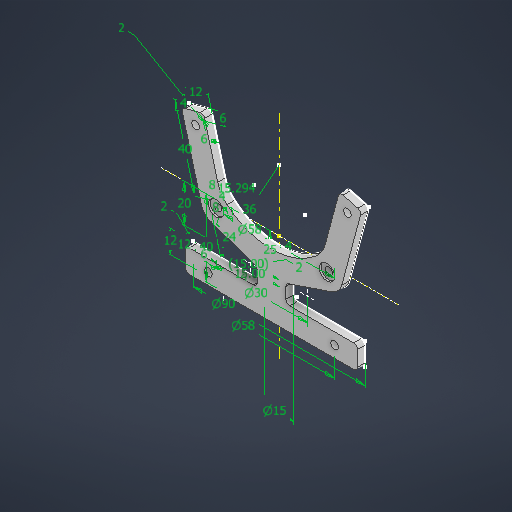
# Autodesk Inventor part: UnitreeGO2_frontmount
Saved by Autodesk Inventor 2026.1 (Build 301233000, 233)
## iProperties
Created: 2026-01-16
Part Number: UnitreeGO2_frontmount
Material: Generic
Document SubType Name: Modeling
Designer: aimot
Density: 1 g/cm^3
Appearance: Default
Author: aimot
Autodesk Inventor part; units mm, degrees
ref_plane "YZ Plane" through (0, 0, 0) normal (1, 0, 0) x (0, 1, 0)
ref_plane "XZ Plane" through (0, 0, 0) normal (0, 1, 0) x (-1, 0, 0)
ref_plane "XY Plane" through (0, 0, 0) normal (0, 0, 1) x (1, 0, 0)
sketch "Sketch1" plane through (0, 0, 0) normal (0, 0, 1) x (1, 0, 0)
  circle A0 centre (-29, 0) radius 2
  line L0 (-62.2888, 0) -> (62.2888, 0) construction
  arc A1 (-36.7274, -2.0706) -> (-31.5768, -7.5737) centre (-29, 0) ccw
  arc A2 (-23.2301, 4.498) -> (0, -4) centre (0, 32) ccw
  line L1 (0, -55.9324) -> (0, 55.5944) construction
  line L2 (-31.5768, -7.5737) -> (-8.8558, -15.304)
  line L3 (-7.5, -17.1974) -> (-7.5, -23)
  line L4 (-36.7274, -2.0706) -> (-46.5625, 34.6346)
  line L5 (-45.1483, 37.0841) -> (-37.4209, 39.1547)
  line L6 (-34.9714, 37.7405) -> (-28.1342, 12.2236)
  arc A3 (-7.5, -17.1974) -> (-8.8558, -15.304) centre (-9.5, -17.1974) ccw
  arc A4 (-45.1483, 37.0841) -> (-46.5625, 34.6346) centre (-44.6307, 35.1523) ccw
  arc A5 (-34.9714, 37.7405) -> (-37.4209, 39.1547) centre (-36.9033, 37.2228) ccw
  circle A6 centre (29, 0) radius 2
  line L7 (62.2888, 0) -> (-62.2888, 0) construction
  arc A7 (31.5768, -7.5737) -> (36.7274, -2.0706) centre (29, 0) ccw
  line L8 (31.5768, -7.5737) -> (8.8558, -15.304)
  line L9 (7.5, -17.1974) -> (7.5, -25)
  line L10 (36.7274, -2.0706) -> (46.5625, 34.6346)
  line L11 (45.1483, 37.0841) -> (37.4209, 39.1547)
  arc A8 (8.8558, -15.304) -> (7.5, -17.1974) centre (9.5, -17.1974) ccw
  arc A9 (46.5625, 34.6346) -> (45.1483, 37.0841) centre (44.6307, 35.1523) ccw
  arc A10 (37.4209, 39.1547) -> (34.9714, 37.7405) centre (36.9033, 37.2228) ccw
  circle A11 centre (-29, 0) radius 4
  circle A12 centre (29, 0) radius 4
  line L12 (-9.5, -25) -> (-43, -25)
  line L13 (-45, -27) -> (-45, -35)
  line L14 (-43, -37) -> (0, -37)
  arc A13 (-43, -25) -> (-45, -27) centre (-43, -27) ccw
  arc A14 (-45, -35) -> (-43, -37) centre (-43, -35) ccw
  arc A15 (-9.5, -25) -> (-7.5, -23) centre (-9.5, -23) ccw
  line L15 (9.5, -25) -> (43, -25)
  line L16 (45, -27) -> (45, -35)
  line L17 (43, -37) -> (0, -37)
  arc A16 (45, -27) -> (43, -25) centre (43, -27) ccw
  arc A17 (43, -37) -> (45, -35) centre (43, -35) ccw
  arc A18 (7.5, -23) -> (9.5, -25) centre (9.5, -23) ccw
  arc A19 (-28.1342, 12.2236) -> (-23.2301, 4.498) centre (-13.3609, 16.1821) ccw
  arc A20 (0, -4) -> (23.2301, 4.498) centre (0, 32) ccw
  line L18 (34.9714, 37.7405) -> (28.1342, 12.2236)
  arc A21 (23.2301, 4.498) -> (28.1342, 12.2236) centre (13.3609, 16.1821) ccw
  circle A22 centre (-39.7317, 32.3238) radius 2
  circle A23 centre (39.7317, 32.3238) radius 2
  circle A24 centre (-33, -31) radius 2
  circle A25 centre (33, -31) radius 2
  point P0 (0, 0)
  point P1 (-7.5, -15.7653)
  point P2 (-47.0802, 36.5665)
  point P3 (-26.9294, 7.7274)
  point P4 (-7.5, -25)
  point P5 (-15, -20)
  point P6 (7.5, -15.7653)
  point P7 (47.0802, 36.5665)
  point P8 (15, -20)
  point P9 (-29, -40)
  point P10 (-45, -25)
  point P11 (-45, -37)
  point P12 (45, -25)
  point P13 (45, -37)
  point P14 (7.5, -23)
  dimension "d0" = 4
  dimension "d1" = 58
  dimension "d7" = 2
  dimension "d9" = 15
  dimension "d12" = 20
  dimension "d13" = 30
  dimension "d15" = 2
  dimension "d19" = 8
  dimension "d20" = 15
  dimension "d21" = 15
  dimension "d22" = 12
  dimension "d24" = 4
  dimension "d26" = 24
  dimension "d28" = 40
  dimension "d40" = 8
  dimension "d45" = 40
  dimension "d46" = 58
  dimension "d47" = 2
  dimension "d48" = 12
  dimension "d49" = 25
  dimension "d50" = 90
  dimension "d53" = 36
  dimension "d54" = 15.2944
  dimension "d55" = 4
  dimension "d56" = 6
  dimension "d57" = 6
  dimension "d61" = 4
  dimension "d62" = 12
  dimension "d63" = 6
  constraints: 40 point on circle, 36 end point, 36 symmetric about line, 26 centre point, 23 point on line, 16 tangent, 4 perpendicular, 3 coincident, 3 equal radius, 1 horizontal, 1 line through centre, 1 vertical, 13 other
  measures "d0" diameter of A0
  measures "d1" diameter of A0.centre L1
  measures "d7" radius of A3
  measures "d9" diameter of L3 L1
  measures "d12" vertical distance of A0.centre point (-15, -20)
  measures "d13" diameter of point (-15, -20) L1
  measures "d15" radius of A4
  measures "d19" radius of A1
  measures "d20" angle of L1 L6
  measures "d21" angle of L1 L4
  measures "d22" distance between parallel lines of L6 L4
  measures "d24" distance from line of L0 A2.end
  measures "d26" distance of L2.start L2.end
  measures "d28" distance from line of A0.centre L5
  measures "d40" diameter of A11
  measures "d45" distance of A0.centre point (-29, -40)
  measures "d46" diameter of point (-29, -40) L1
  measures "d47" radius of A13
  measures "d48" distance between parallel lines of L14 L12
  measures "d49" distance from line of A11.centre L12
  measures "d50" diameter of L13 L1
  measures "d53" radius of A2
  measures "d54" radius of A19
  measures "d55" diameter of A22
  measures "d56" distance from line of L5 A22.centre
  measures "d57" distance from line of L6 A22.centre
  measures "d61" diameter of A24
  measures "d62" distance from line of L13 A24.centre
  measures "d63" distance from line of L12 A24.centre
extrude "Extrusion3" add sketch "Sketch1" along normal blind 3 contours A11 | A12
extrude "Extrusion4" add sketch "Sketch1" along normal blind 4 contours L4 A4 L5 A5 L6 A19 A2 A20 A21 L18 A10 L11 A9 L10 A7 L8 A8 L9 A18 L15 A16 L16 A17 L17 L14 A14 L13 A13 L12 A15 L3 A3 L2 A1
body "Solid2"
